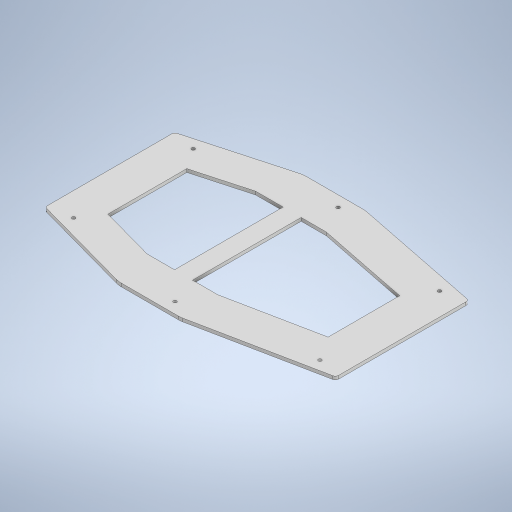
# Autodesk Inventor part: gora
Saved by Autodesk Inventor 2023 (Build 270158000, 158)
## iProperties
Created: 2024-06-29
Part Number: gora
Material: Ogólny
Document SubType Name: Modeling
Designer: kamil
Density: 1 g/cm^3
Appearance: Domyślna
Author: kamil
Autodesk Inventor part; units mm, degrees
ref_plane "YZ Plane" through (0, 0, 0) normal (1, 0, 0) x (0, 1, 0)
ref_plane "XZ Plane" through (0, 0, 0) normal (0, 1, 0) x (-1, 0, 0)
ref_plane "XY Plane" through (0, 0, 0) normal (0, 0, 1) x (1, 0, 0)
sketch "Szkic1" plane through (0, 0, 0) normal (0, 1, 0) x (-1, 0, 0)
  line L0 (-135, 0) -> (135, 0) construction
  line L1 (0, 75) -> (0, -75) construction
  line L2 (0, 75) -> (113.2475, 55)
  line L3 (113.2475, 55) -> (113.2475, -55)
  line L4 (113.2475, -55) -> (0, -75)
  line L5 (-113.2475, -55) -> (-113.2475, 55)
  line L6 (-113.2475, 55) -> (0, 75)
  line L7 (0, -75) -> (-113.2475, -55)
  line L8 (-113.2475, 55) -> (-135, 51.1584)
  line L9 (-135, 51.1584) -> (-135, -51.1584)
  line L10 (-135, -51.1584) -> (-113.2475, -55)
  line L11 (113.2475, 55) -> (135, 51.1584)
  line L12 (113.2475, -55) -> (135, -51.1584)
  line L13 (135, 51.1584) -> (135, -51.1584)
  line L14 (114.9866, -64.8476) -> (145, -59.5471)
  line L15 (145, -59.5471) -> (145, 59.5471)
  line L16 (145, 59.5471) -> (114.9866, 64.8476)
  line L17 (114.9866, 64.8476) -> (0, 85.1547)
  line L18 (0, 85.1547) -> (-114.9866, 64.8476)
  line L19 (-114.7917, -64.882) -> (-145, -59.5471)
  line L20 (-145, -59.5471) -> (-145, 59.5471)
  line L21 (-145, 59.5471) -> (-114.9866, 64.8476)
  line L22 (-114.7917, -64.882) -> (0, -85.1547)
  line L23 (0, -85.1547) -> (114.9866, -64.8476)
  point P0 (0, 0)
  point P1 (0, 0)
  point P2 (0, 0)
  point P3 (135, 0)
  point P4 (-135, 0)
  dimension "d0" = 270
  dimension "d1" = 115
  dimension "d2" = 115
  dimension "d3" = 115
  dimension "d4" = 115
  dimension "d5" = 150
  dimension "d6" = 110
  dimension "d7" = 10
  dimension "d8" = 10
  dimension "d9" = 10
  dimension "d10" = 10
  constraints: 48 end point, 5 vertical, 4 coincident, 4 collinear, 4 midpoint, 4 vertical alignment, 3 horizontal alignment, 1 horizontal, 6 other
  measures "d0" distance of L0.start L0.end
  measures "d1" distance of L1.start L2.end
  measures "d2" distance of L1.end L3.end
  measures "d3" distance of L1.end L5.start
  measures "d4" distance of L1.start L5.end
  measures "d5" distance of L1.end L1.start
  measures "d6" distance of L3.end L2.end
  measures "d7" distance between parallel lines of L13 L15
  measures "d8" distance between parallel lines of L2 L17
  measures "d9" distance between parallel lines of L9 L20
  measures "d10" distance between parallel lines of L7 L22
extrude "Wyciągnięcie proste1" add sketch "Szkic1" along normal blind 3 contours L2 L3 L4 L7 L5 L6 | L11 L13 L12 L3 | L5 L10 L9 L8 | L23 L22 L19 L20 L21 L18 L17 L16 L15 L14
hole "Otwór1" at (-113.2475, 0, 55) at (0, 0, 75) at (113.2475, 0, 55) at (-113.2475, 0, -55) at (0, 0, -75) at (113.2475, 0, -55) direction (0, 1, 0) diameter 3 depth 10 tip angle 118
sketch "Szkic2" plane through (0, 3, 0) normal (0, 1, 0) x (1, 0, 0)
  line L0 (-145, -59.5471) -> (0, -85.1547) projected
  line L1 (0, -85.1547) -> (145, -59.5471) projected
  line L2 (145, 59.5471) -> (0, 85.1547) projected
  line L3 (0, 85.1547) -> (-145, 59.5471) projected
  line L4 (-27.6975, -84.6887) -> (27.6975, -84.6887)
  line L5 (-26.7514, 84.6887) -> (26.7514, 84.6887)
  point P0 (0, 0)
  point P1 (0, 84.6887)
  point P2 (0, -84.6887)
  point P3 (-2.6387, 84.6887)
  point P4 (2.6387, 84.6887)
  point P5 (2.6387, -84.6887)
  point P6 (-2.6387, -84.6887)
  dimension "d20" = 0.466
  dimension "d21" = 0.466
  constraints: 4 end point, 2 horizontal, 2 midpoint, 2 vertical alignment
  measures "d20" distance from line of L4 L0.end
  measures "d21" distance from line of L5 L2.end
extrude "Wyciągnięcie proste2" cut sketch "Szkic2" against normal blind 3
sketch "Szkic3" plane through (0, 0, 0) normal (0, -1, 0) x (1, 0, 0)
  line L0 (-54, -85) -> (19, -85) projected
  line L1 (-141.3381, -18.5594) -> (-148.4685, -58.9346) projected
  line L2 (148.4685, -58.9346) -> (141.3381, -18.5594) projected
  line L3 (-54, -85) -> (-148.4685, -58.9346)
  line L4 (19, -85) -> (148.4685, -58.9346)
  line L5 (148.4685, -58.9346) -> (148.4685, 0)
  line L6 (145, 59.5471) -> (145, -59.5471) projected
  line L7 (-148.4685, -58.9346) -> (-148.4685, 0)
  line L8 (-148.4685, 0) -> (148.4685, 0)
  line L9 (-145, -59.5471) -> (-145, 59.5471) projected
  line L10 (-54, 85) -> (19, 85)
  line L11 (-54, 85) -> (-148.4685, 58.9346)
  line L12 (19, 85) -> (148.4685, 58.9346)
  line L13 (148.4685, 58.9346) -> (148.4685, 0)
  line L14 (-148.4685, 58.9346) -> (-148.4685, 0)
  line L15 (-145, 59.5471) -> (-2.6387, 84.6887) projected
  line L16 (2.6387, 84.6887) -> (145, 59.5471) projected
  line L17 (-2.6387, -84.6887) -> (-145, -59.5471) projected
  line L18 (145, -59.5471) -> (2.6387, -84.6887) projected
  line L19 (-2.6387, -84.6887) -> (2.6387, -84.6887) projected
  line L20 (2.6387, 84.6887) -> (-2.6387, 84.6887) projected
  point P0 (0, 0)
  point P1 (145, 0)
  constraints: 20 end point, 4 symmetric about line, 2 horizontal alignment, 2 vertical, 1 midpoint, 1 perpendicular
extrude "Wyciągnięcie proste3" add sketch "Szkic3" against normal blind 3 contours L3 L1 L9 L17 L19 L18 L6 L2 L4 L0 | L7 L8 L9 L1 | L2 L6 L8 L5 | L14 L11 L10 L12 L13 L8 L6 L16 L20 L15 L9
sketch "Szkic4" plane through (0, 3, 0) normal (0, 1, 0) x (1, 0, 0)
  line L0 (133.8474, 61.0533) -> (126.7423, 25.7615) projected
  line L1 (133.8474, -61.0533) -> (126.7423, -25.7615) projected
  line L2 (-134.2229, 59.5862) -> (-124.6477, 24.883) projected
  line L3 (-134.2229, -59.5862) -> (-124.6477, -24.883) projected
  line L4 (-54, 85) -> (-148.4685, 58.9346) projected
  line L5 (-148.4685, 58.9346) -> (-148.4685, -58.9346) projected
  line L6 (-148.4685, -58.9346) -> (-54, -85) projected
  line L7 (-54, -85) -> (19, -85) projected
  line L8 (19, -85) -> (148.4685, -58.9346) projected
  line L9 (148.4685, -58.9346) -> (148.4685, 58.9346) projected
  line L10 (148.4685, 58.9346) -> (19, 85) projected
  line L11 (19, 85) -> (-54, 85) projected
  circle A0 centre (0, 75) radius 1.5 projected
  circle A1 centre (113.2475, -55) radius 1.5 projected
  circle A2 centre (-113.2475, -55) radius 1.5 projected
  circle A3 centre (0, -75) radius 1.5 projected
  circle A4 centre (-113.2475, 55) radius 1.5 projected
  circle A5 centre (113.2475, 55) radius 1.5 projected
  line L12 (-134.2229, 59.5862) -> (-135.0636, 62.6332)
  line L13 (-134.2229, -59.5862) -> (-135.0636, -62.6332)
  line L14 (133.8474, 61.0533) -> (134.007, 61.846)
  line L15 (133.8474, -61.0533) -> (134.007, -61.846)
  line L16 (134.007, -61.846) -> (134.007, 61.846)
  line L17 (-135.0636, 62.6332) -> (-135.0636, -62.6332)
  point P0 (0, 0)
  constraints: 12 end point, 4 point on line, 3 collinear, 1 parallel, 1 perpendicular, 1 vertical
extrude "Wyciągnięcie proste4" cut sketch "Szkic4" against normal blind 3 contours L17 L6 L5 L4 | L10 L9 L8 L16
sketch "Szkic5" plane through (0, 0, 0) normal (0, -1, 0) x (1, 0, 0)
  line L0 (134.007, 61.846) -> (19, 85) projected
  line L1 (134.007, -61.846) -> (134.007, 61.846) projected
  line L2 (19, -85) -> (134.007, -61.846) projected
  line L3 (-54, -85) -> (19, -85) projected
  line L4 (-135.0636, -62.6332) -> (-54, -85) projected
  line L5 (-135.0636, 62.6332) -> (-135.0636, -62.6332) projected
  line L6 (-54, 85) -> (-135.0636, 62.6332) projected
  line L7 (19, 85) -> (-54, 85) projected
  line L8 (15.1367, 58.236) -> (107.007, 39.7401)
  line L9 (107.007, 39.7401) -> (107.007, -39.7401)
  line L10 (107.007, -39.7401) -> (15.1367, -58.236)
  line L11 (-51.9686, -58.236) -> (-108.7234, -42.5764)
  line L12 (-108.7234, -42.5764) -> (-108.7234, 42.5764)
  line L13 (-108.7234, 42.5764) -> (-51.9686, 58.236)
  line L14 (-17.2318, 58.236) -> (-17.2318, -58.236)
  line L15 (-17.2318, 58.236) -> (15.1367, 58.236)
  line L16 (15.1367, -58.236) -> (-17.2318, -58.236)
  line L17 (-2.2318, -43.236) -> (-2.2318, 43.236)
  line L18 (-2.2318, 43.236) -> (13.6417, 43.236)
  line L19 (13.6417, 43.236) -> (92.007, 27.459)
  line L20 (92.007, 27.459) -> (92.007, -27.459)
  line L21 (92.007, -27.459) -> (13.6417, -43.236)
  line L22 (13.6417, -43.236) -> (-2.2318, -43.236)
  line L23 (-51.9686, 58.236) -> (-17.2318, 58.236)
  line L24 (-17.2318, -58.236) -> (-51.9686, -58.236)
  line L25 (-17.2318, 43.236) -> (-49.9372, 43.236)
  line L26 (-49.9372, 43.236) -> (-93.7234, 31.1547)
  line L27 (-93.7234, 31.1547) -> (-93.7234, -31.1547)
  line L28 (-93.7234, -31.1547) -> (-49.9372, -43.236)
  line L29 (-49.9372, -43.236) -> (-17.2318, -43.236)
  line L30 (-32.2318, 70) -> (-32.2318, -70)
  point P0 (0, 0)
  point P1 (-32.2318, -43.236)
  point P2 (-32.2318, 43.236)
  dimension "d28" = 27
  dimension "d29" = 15
  dimension "d30" = 15
  dimension "d31" = 15
  constraints: 46 end point, 5 parallel, 1 horizontal, 1 perpendicular, 13 other
  measures "d28" distance between parallel lines of L0 L8
  measures "d29" distance between parallel lines of L14 L17
  measures "d30" distance between parallel lines of L23 L25
  measures "d31" distance between parallel lines of L14 L30
extrude "Wyciągnięcie proste5" cut sketch "Szkic5" against normal blind 3 contours L30 L29 L28 L27 L26 L25 | L17 L18 L19 L20 L21 L22
sketch "Szkic6" plane through (0, 3, 0) normal (0, 1, 0) x (1, 0, 0)
  line L0 (62.2834, -75.4611) -> (133.8474, -61.0533) projected
  line L1 (-135.0636, -59.3542) -> (-42.1161, -85) projected
  line L2 (62.2834, 75.4611) -> (133.8474, 61.0533) projected
  line L3 (-135.0636, 59.3542) -> (-42.1161, 85) projected
  line L4 (-54, -85) -> (19, -85) projected
  line L5 (19, -85) -> (134.007, -61.846) projected
  line L6 (62.2834, -75.4611) -> (14.903, -85)
  line L7 (134.007, 61.846) -> (19, 85) projected
  line L8 (19, 85) -> (-54, 85) projected
  line L9 (-135.0636, 62.6332) -> (-135.0636, -62.6332) projected
  line L10 (-135.0636, -62.6332) -> (-54, -85) projected
  line L11 (-54, 85) -> (-135.0636, 62.6332) projected
  line L12 (134.007, -61.846) -> (134.007, 61.846) projected
  line L13 (62.2834, 75.4611) -> (14.903, 85)
  line L14 (133.8474, 61.0533) -> (134.007, 61.0212)
  line L15 (133.8474, -61.0533) -> (134.007, -61.0212)
  point P0 (0, 0)
  constraints: 8 end point, 4 point on line, 2 collinear, 2 parallel
extrude "Wyciągnięcie proste6" cut sketch "Szkic6" against normal through all contours L0 L15 L12 L5 L4 L6 | L4 L10 L9 L1 | L14 L2 L13 L8 L7 L12 | L9 L11 L8 L3
sketch "Szkic7" plane through (0, 3, 0) normal (0, 1, 0) x (1, 0, 0)
  line L0 (13.6417, 43.236) -> (92.007, 27.459) projected
  line L1 (-2.2318, 43.236) -> (13.6417, 43.236) projected
  line L2 (-2.2318, -43.236) -> (-2.2318, 43.236) projected
  line L3 (92.007, -27.459) -> (13.6417, -43.236) projected
  line L4 (13.6417, -43.236) -> (-2.2318, -43.236) projected
  line L5 (92.007, 27.459) -> (92.007, -27.459) projected
  line L6 (-32.2318, 43.236) -> (-32.2318, -43.236) projected
  line L7 (-49.9372, 43.236) -> (-32.2318, 43.236) projected
  line L8 (-93.7234, 31.1547) -> (-49.9372, 43.236) projected
  line L9 (-93.7234, -31.1547) -> (-93.7234, 31.1547) projected
  line L10 (-49.9372, -43.236) -> (-93.7234, -31.1547) projected
  line L11 (-32.2318, -43.236) -> (-49.9372, -43.236) projected
  line L12 (-50.8456, 49.944) -> (-25.5238, 49.944)
  line L13 (-25.5238, 49.944) -> (-25.5238, -49.944)
  line L14 (-25.5238, -49.944) -> (-50.8456, -49.944)
  line L15 (-50.8456, -49.944) -> (-100.4314, -36.2625)
  line L16 (-100.4314, -36.2625) -> (-100.4314, 36.2625)
  line L17 (-100.4314, 36.2625) -> (-50.8456, 49.944)
  line L18 (14.3102, 49.944) -> (98.715, 32.9511)
  line L19 (98.715, 32.9511) -> (98.715, -32.9511)
  line L20 (98.715, -32.9511) -> (14.3102, -49.944)
  line L21 (14.3102, -49.944) -> (-8.9398, -49.944)
  line L22 (-8.9398, -49.944) -> (-8.9398, 49.944)
  line L23 (-8.9398, 49.944) -> (14.3102, 49.944)
  point P0 (0, 0)
  dimension "d36" = 6.708
  dimension "d37" = 6.708
  constraints: 24 end point, 10 other
  measures "d36" distance between parallel lines of L13 L6
  measures "d37" distance between parallel lines of L2 L22
extrude "Wyciągnięcie proste7" cut sketch "Szkic7" against normal through all contours L0 L5 L3 L4 L2 L1 | L6 L11 L10 L9 L8 L7 | L12 L13 L14 L15 L16 L17 | L18 L19 L20 L21 L22 L23
fillet "Zaokrąglenie1" radius 20 4 edges at (-42.1161, 1.5, 85) (14.903, 1.5, 85) (-42.1161, 1.5, -85) (14.903, 1.5, -85)
fillet "Zaokrąglenie2" radius 3 4 edges at (134.007, 1.5, 61.0212) (134.007, 1.5, -61.0212) (-135.0636, 1.5, 59.3542) (-135.0636, 1.5, -59.3542)
